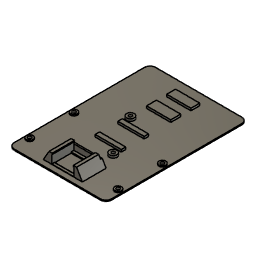
Component plate v6 (Autodesk Fusion 360 design; units mm, degrees)
Autodesk Fusion 360 part; units mm, degrees
sketch "Sketch1" plane through (0, 0, 0) normal (0, 1, 0) x (1, 0, 0)
  line L0 (-33.5, 76.6) -> (-54.5, 76.6) construction
  line L1 (-54.5, 76.6) -> (-54.5, 40) construction
  line L2 (-54.5, 40) -> (-33.5, 40) construction
  line L3 (-33.5, 40) -> (-33.5, 76.6) construction
  circle A0 centre (-33.5, 40) radius 1.5
  circle A1 centre (-54.5, 76.6) radius 1.5
  line L4 (0, 0) -> (-88, 0)
  line L5 (-88, 0) -> (-88, 127.8)
  line L6 (-88, 127.8) -> (0, 127.8)
  line L7 (0, 127.8) -> (0, 0)
  line L8 (-44, 40) -> (-44, 0) construction
  line L9 (-33.05, 91.6) -> (-54.95, 91.6)
  line L10 (-54.95, 91.6) -> (-54.95, 117.8)
  line L11 (-54.95, 117.8) -> (-33.05, 117.8)
  line L12 (-33.05, 117.8) -> (-33.05, 91.6)
  line L13 (-44, 91.6) -> (-44, 76.6) construction
  line L14 (-33.05, 100.6) -> (-54.95, 100.6)
  line L15 (-33.05, 109.8) -> (-54.95, 109.8)
  circle A2 centre (-33.5, 40) radius 3.5
  circle A3 centre (-54.5, 76.6) radius 3.5
  line L16 (-32.15, 46) -> (-55.85, 46)
  line L17 (-55.85, 46) -> (-55.85, 70.6)
  line L18 (-55.85, 70.6) -> (-32.15, 70.6)
  line L19 (-32.15, 70.6) -> (-32.15, 46)
  line L20 (-32.15, 50) -> (-55.85, 50)
  line L21 (-32.15, 66.6) -> (-55.85, 66.6)
  line L22 (-44, 40) -> (-44, 46) construction
  line L23 (-32.15, 58.3) -> (-33.5, 58.3) construction
  circle A4 centre (-84, 15) radius 1.6
  circle A5 centre (-4, 15) radius 1.6
  line L24 (-84, 15) -> (-84, 55) construction
  circle A6 centre (-84, 55) radius 1.6
  circle A7 centre (-4, 55) radius 1.6
  circle A8 centre (-84, 15) radius 3.1
  circle A9 centre (-84, 55) radius 3.1
  circle A10 centre (-4, 55) radius 3.1
  circle A11 centre (-4, 15) radius 3.1
  line L25 (-54, 25) -> (-34, 25)
  line L26 (-34, 25) -> (-34, 5)
  line L27 (-34, 5) -> (-54, 5)
  line L28 (-54, 5) -> (-54, 25)
  line L29 (-54, 25) -> (-57, 25)
  line L30 (-57, 25) -> (-57, 5)
  line L31 (-57, 5) -> (-54, 5)
  line L32 (-34, 25) -> (-31, 25)
  line L33 (-31, 25) -> (-31, 5)
  line L34 (-31, 5) -> (-34, 5)
  line L35 (-54, 22.5) -> (-34, 22.5)
  line L36 (-54, 15) -> (-34, 15) construction
  line L37 (-54, 7.5) -> (-34, 7.5)
  line L38 (-53.5, 25) -> (-53.5, 5)
  line L39 (-34.5, 25) -> (-34.5, 5)
  line L40 (-64.248, 0) -> (-21.8626, 0)
  line L41 (-21.8626, 0) -> (-21.8626, 29.5864)
  line L42 (-21.8626, 29.5864) -> (-64.248, 29.5864)
  line L43 (-64.248, 29.5864) -> (-64.248, 0)
  line L44 (-57, 25) -> (-57, 26.5)
  line L45 (-57, 26.5) -> (-31, 26.5)
  line L46 (-31, 26.5) -> (-31, 25)
  dimension "d1" = 36.6
  dimension "d2" = 21
  dimension "d3" = 3
  dimension "d4" = 88
  dimension "d6" = 21.9
  dimension "d7" = 26.2
  dimension "d8" = 15
  dimension "d9" = 9
  dimension "d10" = 8
  dimension "d11" = 2
  dimension "d13" = 10
  dimension "d21" = 23.7
  dimension "d22" = 4
  dimension "d23" = 4
  dimension "d24" = 6
  dimension "d25" = 80
  dimension "d26" = 3.2
  dimension "d27" = 40
  dimension "d29" = 0.5
  dimension "d31" = 3
  dimension "d32" = 15
  dimension "d34" = 5
  dimension "d35" = 20
  dimension "d57" = 1.5
  dimension "d60" = 15
  dimension "d63" = 1.5
  constraint horizontal L0
  constraint vertical L1
  constraint horizontal L2
  constraint vertical L3
  constraint coincident L2.end L3.start
  constraint coincident L0.end L1.start
  constraint equal A0 A1
  constraint horizontal L4
  constraint vertical L5
  constraint horizontal L6
  constraint vertical L7
  constraint coincident L4.start L7.end
  constraint midpoint L2 L8.start
  constraint midpoint L4 L8.end
  constraint vertical L8
  constraint horizontal L9
  constraint vertical L10
  constraint horizontal L11
  constraint vertical L12
  constraint midpoint L9 L13.start
  constraint midpoint L0 L13.end
  constraint vertical L13
  constraint coincident L12 L14.start
  constraint coincident L10 L14.end
  constraint perpendicular L10 L14
  constraint coincident L12 L15.start
  constraint coincident L10 L15.end
  constraint perpendicular L10 L15
  constraint concentric A1 A3
  constraint equal A2 A3
  constraint horizontal L16
  constraint vertical L17
  constraint horizontal L18
  constraint vertical L19
  constraint coincident L19 L20.start
  constraint coincident L17 L20.end
  constraint perpendicular L17 L20
  constraint coincident L19 L21.start
  constraint coincident L17 L21.end
  constraint perpendicular L17 L21
  constraint midpoint L16 L22.end
  constraint midpoint L19 L23.start
  constraint midpoint L3 L23.end
  constraint vertical L22
  constraint horizontal L23
  constraint symmetric L8 A4 A5
  constraint coincident A4.centre L24.start
  constraint vertical L24
  constraint coincident L24.end A6.centre
  constraint symmetric L22 A6 A7
  constraint equal A4 A6
  constraint equal A8 A9
  constraint symmetric L8 A8 A11
  constraint symmetric L8 A9 A10
  constraint horizontal L25
  constraint vertical L26
  constraint horizontal L27
  constraint vertical L28
  constraint perpendicular L28 L29
  constraint perpendicular L27 L30
  constraint perpendicular L28 L31
  constraint perpendicular L26 L32
  constraint perpendicular L27 L33
  constraint perpendicular L26 L34
  constraint coincident L28 L35.start
  constraint coincident L26 L35.end
  constraint perpendicular L26 L35
  constraint midpoint L28 L36.start
  constraint midpoint L26 L36.end
  constraint coincident L28 L37.start
  constraint coincident L26 L37.end
  constraint perpendicular L28 L37
  constraint coincident L25 L38.start
  constraint coincident L27 L38.end
  constraint perpendicular L27 L38
  constraint coincident L27 L39.end
  constraint perpendicular L35 L39
  constraint symmetric L8 L38 L39
  constraint symmetric L35 L36 L37
  constraint coincident L25 L39.start
  constraint equal L27 L28
  constraint coincident A4.centre L36
  constraint horizontal L40
  constraint vertical L41
  constraint horizontal L42
  constraint vertical L43
  constraint coincident L4 L40.start
  constraint perpendicular L29 L44
  constraint perpendicular L26 L45
  constraint perpendicular L45 L46
  measures "d1" distance of L0.end L1.end
  measures "d2" distance of L0.start L0.end
  measures "d3" diameter of A0
  measures "d4" distance of L4.start L4.end
  measures "d6" distance of L9.start L9.end
  measures "d7" distance of L9.start L11.end
  measures "d8" distance of L13.start L13.end
  measures "d9" distance of L9 L14
  measures "d10" distance of L11 L15
  measures "d13" distance of L6 L11
  measures "d21" distance of L16.start L16.end
  measures "d22" distance of L16 L20
  measures "d23" distance of L18 L21
  measures "d24" distance of L2 L16
  measures "d25" distance of A4.centre A5.centre
  measures "d26" diameter of A4
  measures "d27" distance of A4.centre L24.end
  measures "d29" distance of L26 L39
  measures "d31" distance of L25.end L32.end
  measures "d32" distance of L2.end L25
  measures "d34" distance of L4 L34
  measures "d35" distance of L25.start L27.end
  measures "d57" distance of A4 A8
  measures "d60" distance of L35 L37
  measures "d63" distance of L29.end L44.end
extrude "Extrude1" add sketch "Sketch1" against normal blind 1 contours L4 L5 L6 L7 L41 L42 L43 | L4 L40 L41 L42 L43 | L9 L10 L12 L14 | L10 L12 L14 L15 | L10 L11 L12 L15 | A2 | A3 | L16 L17 L19 L20 | L17 L19 L20 L21 | L17 L18 L19 L21 | A4 | A5 | A6 | A7 | A8 | A9 | A10 | A11 | L25 L29 L32 L44 L45 L46 | L25 L28 L35 L38 | L28 L29 L30 L31 | L25 L35 L38 L39 | L28 L35 L37 L38 | L25 L26 L35 L39 | L35 L37 L38 L39 | L27 L28 L37 L38 | L26 L32 L33 L34 | L26 L35 L37 L39 | L27 L37 L38 L39 | L26 L27 L37 L39
extrude "Extrude2" add sketch "Sketch1" along normal blind 2 contours L9 L10 L12 L14 | L10 L11 L12 L15
extrude "Extrude3" add sketch "Sketch1" along normal blind 3 from surface at -1 contours A2 | A3 | L16 L17 L19 L20 | L17 L18 L19 L21
extrude "Extrude4" add sketch "Sketch1" along normal blind 8 contours L28 L29 L30 L31 | L26 L32 L33 L34
extrude "Extrude5" add sketch "Sketch1" along normal blind 1 from surface at 8 contours L25 L28 L35 L38 | L28 L29 L30 L31 | L28 L35 L37 L38 | L25 L26 L35 L39 | L27 L28 L37 L38 | L26 L32 L33 L34 | L26 L35 L37 L39 | L26 L27 L37 L39
extrude "Extrude6" add sketch "Sketch1" along normal blind 1 contours L25 L28 L35 L38 | L25 L35 L38 L39 | L25 L26 L35 L39
extrude "Extrude7" add sketch "Sketch1" along normal blind 0.3 contours L27 L28 L37 L38 | L27 L37 L38 L39 | L26 L27 L37 L39
extrude "Extrude11" add sketch "Sketch1" along normal blind 6 contours L25 L29 L32 L44 L45 L46
draft "Draft1" angle -30 neutral plane through (0, 8, 0) pull (0, -1, 0) 1 faces at (-57, 3, -11.6667)
draft "Draft2" angle -30 neutral plane through (0, 8, 0) pull (0, -1, 0) 1 faces at (-31, 3, -18.3333)
draft "Draft3" angle 30 neutral plane through (-53.5, 8, -7.5) pull (1, 0, 0) 1 faces at (-53.6667, 8, -18.3333)
draft "Draft4" angle 30 neutral plane through (-34.5, 8, -25) pull (-1, 0, 0) 1 faces at (-34.3333, 8, -18.3333)
extrude "Extrude8" cut sketch "Sketch1" against normal up to surface (1 mm away) contours A4 | A5 | A6 | A7
extrude "Extrude9" add sketch "Sketch1" along normal blind 1 contours A8 | A9 | A10 | A11
fillet "Fillet1" radius 5 4 edges at (0, -0.5, 0) (-88, -0.5, 0) (0, -0.5, -127.8) (-88, -0.5, -127.8)
extrude "Extrude10" [suppressed]
equation "d4 = 90 mm - 2 mm"
equation "d23 = d22"
named bodies: "Component plate"
